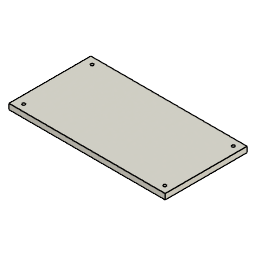
ATN Holder (Autodesk Fusion 360 design; units mm, degrees)
part number: 2026-03-09-17-59-10-170
Autodesk Fusion 360 part; units mm, degrees
sketch "Sketch1" plane through (0, 0, 0) normal (0, 0, 1) x (1, 0, 0)
  line L0 (0, 0) -> (112.014, 0)
  line L1 (112.014, 0) -> (112.014, 58.741)
  line L2 (112.014, 58.741) -> (0, 58.741)
  line L3 (0, 58.741) -> (0, 0)
  circle A0 centre (106.934, 4.826) radius 1.016
  circle A1 centre (5.8, 4.826) radius 1.016
  circle A2 centre (5.8, 53.915) radius 1.016
  circle A3 centre (106.934, 53.915) radius 1.016
  dimension "d1" = 112.014
  dimension "d2" = 58.741
  dimension "d3" = 2.032
  dimension "d4" = 2.032
  dimension "d5" = 2.032
  dimension "d6" = 2.032
  constraint horizontal L0
  constraint vertical L1
  constraint horizontal L2
  constraint vertical L3
  constraint coincident L0.start L3.end
  measures "d1" distance of L0.start L0.end
  measures "d2" distance of L0.start L2.end
  measures "d3" diameter of A0
  measures "d4" diameter of A1
  measures "d5" diameter of A2
  measures "d6" diameter of A3
extrude "Extrude1" add sketch "Sketch1" along normal blind 4
